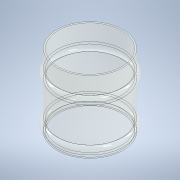
# Autodesk Inventor part: Tubo Corrugado 22mm
Saved by Autodesk Inventor 2020.3 (Build 243373000, 373)
## iProperties
Created: 2020-07-11
Part Number: Tubo Corrugado 22mm
Material: Glass
Document SubType Name: Modeling
Designer: Bruno
Density: 2.18 g/cm^3
Appearance: Clear
Author: Bruno
Autodesk Inventor part; units mm, degrees
ref_plane "YZ Plane" through (0, 0, 0) normal (1, 0, 0) x (0, 1, 0)
ref_plane "XZ Plane" through (0, 0, 0) normal (0, 1, 0) x (-1, 0, 0)
ref_plane "XY Plane" through (0, 0, 0) normal (0, 0, 1) x (1, 0, 0)
sketch "Sketch2" plane through (0, 0, 0) normal (1, 0, 0) x (0, 1, 0)
  line L0 (0, 11.5) -> (1, 11.5)
  line L1 (4, 11.5) -> (16, 11.5)
  line L2 (19, 11.5) -> (25, 11.5)
  arc A0 (19, 11.5) -> (16, 11.5) centre (17.5, 10.875) ccw
  arc A1 (4, 11.5) -> (1, 11.5) centre (2.5, 10.875) ccw
  line L3 (25, 11) -> (18.618, 11)
  arc A2 (18.618, 11) -> (16.382, 11) centre (17.5, 10.875) ccw
  line L4 (16.382, 11) -> (3.618, 11)
  arc A3 (3.618, 11) -> (1.382, 11) centre (2.5, 10.875) ccw
  line L5 (1.382, 11) -> (0, 11)
  line L6 (0, 11.5) -> (0, 11)
  line L7 (25, 11.5) -> (25, 11)
  line L8 (0, 0) -> (2.8216, 0)
  dimension "d1" = 11.5
  dimension "d5" = 12
  dimension "d9" = 6
  dimension "d11" = 1.625
  dimension "d12" = 1.625
  dimension "d13" = 1
  dimension "d14" = 11.5
  dimension "d15" = 0.5
  constraints: 18 end point, 8 point on circle, 4 centre point, 2 horizontal, 1 parallel, 1 vertical, 4 other
  measures "d1" distance from line of L8.start L0
  measures "d5" distance of L1.start L1.end
  measures "d9" distance of L2.start L2.end
  measures "d11" radius of A1
  measures "d12" radius of A0
  measures "d13" distance of L0.start L0.end
  measures "d14" distance from line of L8.start L1
  measures "d15" distance between parallel lines of L1 L4
revolve "Revolution1" add sketch "Sketch2" angle 360 about axis through (0, 0, 0) along (0, 1, 0)
body "Solid1"
